Autodesk Fusion 360 part; units mm, degrees
(part 2 of 2)
extrude "Extrude1'" add sketch "clean_plate_v4.1" along normal blind 3 separate body contours L0 L1 L2 L3 L4 L5 A0 L29 L30 L33 L34 L36 L39 L40 L42 L43 L44 L46 L50 L51 L52 L53 L54 A2 L281 A12 L282 L283 L367 L368 L369 L370 A16 L371 L373 L374 L375 L377 L378 L379 L380 L381 L382 L383 L384 L386 L387 L390 L391 L392 L393 L395 L396 A17 L398 L399 L400 L403 L404 | L6 L7 L28 L31 L32 L41 A1 L64 L72 A4 L124 L126 L131 L133 L135 L136 L141 L142 L143 L144 L151 L154 L155 L157 L159 L160 L161 L166 L167 L169 L170 L171 L173 L174 L179 L181 L184 L185 L187 L188 L190 L192 L194 L195 L198 L200 L201 L204 L205 L208 L210 L215 L219 L225 L231 A13 A14 A15 | L8 L9 L15 L27 | L10 L12 L17 L21 | L11 L23 L24 L25 | L13 L14 L385 L397 | L16 L18 L19 L22 | L20 L127 L148 L156 | L26 L97 L115 L120 | L35 L376 L401 L402 | L37 L45 L49 L394 | L38 L55 L372 L389 | L47 L48 L56 L388 | L57 L74 L77 L363 | L58 L81 L355 L364 | L59 L253 L254 L257 | L60 L68 L91 L366 | L61 L65 L308 L310 | L62 L69 L80 L365 | L63 L246 L252 L256 | L66 L73 L82 L306 | L67 L70 L79 L85 | A3 | A9 | A7 | A5 | L260 L261 L262 L263 L264 L265 L267 L270 L274 L275 L276 L277 L278 L279 L280 L284 L285 L286 L287 L288 L289 L290 L291 L292 L293 L294 L295 L297 L298 L300 L301 L303 L304 L309 L311 L312 L314 L316 L318 L319 L321 L322 L323 L324 L325 L327 L329 L330 L331 L332 L335 L337 L338 L339 L342 L343 L345 L347 | L71 L75 L88 L353 | L76 L78 L83 L350 | L84 L86 L87 L90 | L89 L92 L357 L358 | L93 L94 L103 L104 | L95 L129 L130 L139 | L96 L106 L113 L116 | L98 L99 L102 L117 | L100 L108 L111 L118 | L101 L112 L121 L122 | L105 L107 L110 L114 | L109 L128 L137 L153 | L119 L123 L132 L140 | L125 L134 L180 L189 | L138 L147 L150 L152 | L145 L146 L149 L269 | L158 L175 L202 L207 | L162 L224 L227 L232 | L163 L177 L199 L221 | L164 L165 L172 L182 | L168 L209 L212 L214 | L176 L196 L213 L217 | L178 L211 L216 L230 | L183 L186 L191 L203 | L193 L206 L218 L226 | L197 L220 L222 L223 | L228 L229 L233 L237 | L234 L247 L248 L249 | L235 L236 L238 L250 | L239 L240 L241 L242 | L243 L244 L245 L251 | L255 L258 L259 L305 | L266 L326 L334 L346 | L268 L271 L272 L273 | L296 L317 L320 L340 | L299 L315 L336 L341 | L302 L328 L333 L344 | L307 L313 L356 L362 | L348 L351 L359 L361 | L349 L352 L354 L360 makes body 2 in component "bottom_right"
extrude "Extrude2'" cut sketch "clean_plate_v4.1" along normal blind 10 contours L0 L1 L2 L3 L4 L5 A0 L29 L30 L33 L34 L36 L39 L40 L42 L43 L44 L46 L50 L51 L52 L53 L54 A2 L281 A12 L282 L283 L367 L368 L369 L370 A16 L371 L373 L374 L375 L377 L378 L379 L380 L381 L382 L383 L384 L386 L387 L390 L391 L392 L393 L395 L396 A17 L398 L399 L400 L403 L404 | L6 L7 L28 L31 L32 L41 A1 L64 L72 A4 L124 L126 L131 L133 L135 L136 L141 L142 L143 L144 L151 L154 L155 L157 L159 L160 L161 L166 L167 L169 L170 L171 L173 L174 L179 L181 L184 L185 L187 L188 L190 L192 L194 L195 L198 L200 L201 L204 L205 L208 L210 L215 L219 L225 L231 A13 A14 A15 | A3 | A9 | A7 | A5 bodies 2 in component "bottom_right"
extrude "Extrude3'" add sketch "clean_plate_v4.1" along normal blind 10 contours L0 L1 L2 L3 L4 L5 A0 L29 L30 L33 L34 L36 L39 L40 L42 L43 L44 L46 L50 L51 L52 L53 L54 A2 L281 A12 L282 L283 L367 L368 L369 L370 A16 L371 L373 L374 L375 L377 L378 L379 L380 L381 L382 L383 L384 L386 L387 L390 L391 L392 L393 L395 L396 A17 L398 L399 L400 L403 L404 | L6 L7 L28 L31 L32 L41 A1 L64 L72 A4 L124 L126 L131 L133 L135 L136 L141 L142 L143 L144 L151 L154 L155 L157 L159 L160 L161 L166 L167 L169 L170 L171 L173 L174 L179 L181 L184 L185 L187 L188 L190 L192 L194 L195 L198 L200 L201 L204 L205 L208 L210 L215 L219 L225 L231 A13 A14 A15 | A3 | A9 | A7 | A5 bodies 2 in component "bottom_right"
extrude "Extrude4" cut sketch "clean_plate_v4.1" along normal blind 10 contours L0 L1 L2 L3 L4 L5 A0 L29 L30 L33 L34 L36 L39 L40 L42 L43 L44 L46 L50 L51 L52 L53 L54 A2 L281 A12 L282 L283 L367 L368 L369 L370 A16 L371 L373 L374 L375 L377 L378 L379 L380 L381 L382 L383 L384 L386 L387 L390 L391 L392 L393 L395 L396 A17 L398 L399 L400 L403 L404 | A3 | A9 | A7 | A5 bodies 2 makes body 3 at (77.3381, -75.3022, 10) in component "bottom_right"
extrude "Extrude5" add sketch "clean_plate_v4.1" along normal blind 7 contours L0 L1 L2 L3 L4 L5 A0 L29 L30 L33 L34 L36 L39 L40 L42 L43 L44 L46 L50 L51 L52 L53 L54 A2 L281 A12 L282 L283 L367 L368 L369 L370 A16 L371 L373 L374 L375 L377 L378 L379 L380 L381 L382 L383 L384 L386 L387 L390 L391 L392 L393 L395 L396 A17 L398 L399 L400 L403 L404 | A3 | A9 | A7 | A5 bodies 2 3 in component "bottom_right"
sketch "clean_plate_v4.1 (2)" plane through (0, 0, 0) normal (0, 0, 1) x (1, 0, 0) in component "top_left"
  line L0 (78.2004, -36.6162) -> (78.2605, -36.027)
  line L1 (224.705, -44.1568) -> (224.705, -44.9557)
  line L2 (78.2605, -36.027) -> (78.4684, -35.3561)
  line L3 (79.2324, -34.2221) -> (79.7595, -33.7872)
  arc A0 (179.1936, -126.194) -> (177.1936, -128.1938) centre (179.1936, -128.194) ccw
  line L4 (78.4684, -35.3561) -> (78.798, -34.7487)
  line L5 (78.798, -34.7487) -> (79.2324, -34.2221)
  line L6 (79.7595, -33.7872) -> (80.3665, -33.4582)
  line L7 (80.3665, -33.4582) -> (81.0392, -33.2493)
  line L8 (174.6938, -126.6937) -> (174.693, -134.5617)
  line L9 (98.7866, -145.4708) -> (98.354, -145.6898)
  line L10 (81.6298, -33.1903) -> (171.891, -33.187)
  line L11 (96.953, -145.9308) -> (96.1686, -145.7726)
  line L12 (80.8467, -125.7147) -> (77.5111, -119.9268)
  line L13 (75.6971, -41.0327) -> (75.7005, -36.4881)
  line L14 (224.705, -62.8443) -> (224.705, -102.1057)
  line L15 (171.891, -33.187) -> (218.5412, -40.2054)
  line L16 (78.1951, -43.6543) -> (78.2004, -36.6162)
  line L17 (81.0392, -33.2493) -> (81.6298, -33.1903)
  line L18 (92.4734, -145.8895) -> (89.7788, -141.2137)
  line L19 (75.6449, -110.7467) -> (75.6837, -58.9213)
  arc A1 (222.205, -104.7254) -> (222.205, -117.3746) centre (223.705, -111.05) cw
  line L20 (101.0994, -115.1193) -> (87.243, -123.1193)
  line L21 (98.354, -145.6898) -> (97.7123, -145.8798)
  line L22 (222.205, -44.5066) -> (222.205, -47.5754)
  line L23 (171.498, -138.3375) -> (170.8165, -138.405)
  arc A2 (177.6938, -123.694) -> (174.6938, -126.6937) centre (177.6938, -126.694) ccw
  line L24 (221.5253, -121.9381) -> (221.0349, -122.5329)
  line L25 (221.0885, -41.8996) -> (221.8203, -43.1589)
  line L26 (170.8165, -138.405) -> (110.9915, -138.405)
  line L27 (169.95, -115.8) -> (153.95, -115.8)
  line L28 (172.2545, -138.1006) -> (171.498, -138.3375)
  line L29 (174.6225, -135.2197) -> (174.3886, -135.9665)
  line L30 (96.1686, -145.7726) -> (95.4672, -145.4279)
  line L31 (174.0203, -136.6471) -> (173.5299, -137.2419)
  line L32 (221.8955, -121.2539) -> (221.5253, -121.9381)
  line L33 (174.693, -134.5617) -> (174.6225, -135.2197)
  line L34 (221.8203, -43.1589) -> (222.205, -44.5066)
  line L35 (94.9201, -144.9603) -> (94.5516, -144.4887)
  line L36 (218.5412, -40.2054) -> (219.9033, -40.8617)
  line L37 (219.7584, -123.3922) -> (218.9873, -123.6328)
  line L38 (94.5516, -144.4887) -> (90.6367, -137.6956)
  arc A3 (222.205, -47.5754) -> (222.205, -60.2246) centre (223.705, -53.9) cw
  arc A4 (90.6367, -137.6956) -> (84.3208, -126.7362) centre (86.1791, -132.9649) cw
  line L39 (78.7161, -115.942) -> (78.4204, -114.4636)
  line L40 (222.205, -117.3746) -> (222.205, -119.8357)
  line L41 (134.898, -116.828) -> (134.898, -132.828)
  line L42 (131.85, -134.2) -> (131.85, -118.2)
  line L43 (109.0994, -128.9757) -> (101.0994, -115.1193)
  line L44 (173.5299, -137.2419) -> (172.9351, -137.7323)
  line L45 (150.898, -132.828) -> (150.898, -116.828)
  line L46 (84.3208, -126.7362) -> (79.7448, -118.7959)
  line L47 (115.85, -118.2) -> (115.85, -134.2)
  line L48 (153.95, -131.8) -> (169.95, -131.8)
  line L49 (79.7448, -118.7959) -> (79.0518, -117.2209)
  line L50 (219.9033, -40.8617) -> (221.0885, -41.8996)
  line L51 (110.9915, -138.405) -> (98.7866, -145.4708)
  line L52 (172.9351, -137.7323) -> (172.2545, -138.1006)
  line L53 (95.243, -136.9757) -> (109.0994, -128.9757)
  line L54 (222.1218, -120.5231) -> (221.8955, -121.2539)
  line L55 (220.4401, -123.0233) -> (219.7584, -123.3922)
  line L56 (169.95, -131.8) -> (169.95, -115.8)
  line L57 (87.243, -123.1193) -> (95.243, -136.9757)
  line L58 (218.2905, -123.694) -> (177.6938, -123.694)
  line L59 (78.2135, -111.9846) -> (78.145, -110.6818)
  line L60 (78.145, -110.6818) -> (78.1857, -56.3034)
  line L61 (222.205, -119.8357) -> (222.1218, -120.5231)
  line L62 (222.205, -60.2246) -> (222.205, -104.7254)
  line L63 (79.0518, -117.2209) -> (78.7161, -115.942)
  line L64 (221.0349, -122.5329) -> (220.4401, -123.0233)
  line L65 (78.4204, -114.4636) -> (78.2803, -112.8531)
  arc A5 (78.1857, -56.3034) -> (78.1951, -43.6543) centre (76.6904, -49.9778) cw
  line L66 (218.9873, -123.6328) -> (218.2905, -123.694)
  line L67 (134.898, -132.828) -> (150.898, -132.828)
  line L68 (78.2803, -112.8531) -> (78.2135, -111.9846)
  line L69 (115.85, -134.2) -> (131.85, -134.2)
  line L70 (97.7123, -145.8798) -> (96.953, -145.9308)
  line L71 (174.3886, -135.9665) -> (174.0203, -136.6471)
  line L72 (131.85, -118.2) -> (115.85, -118.2)
  line L73 (95.4672, -145.4279) -> (94.9201, -144.9603)
  line L74 (150.898, -116.828) -> (134.898, -116.828)
  line L75 (153.95, -115.8) -> (153.95, -131.8)
  circle A6 centre (86.1791, -132.9649) radius 2
  line L76 (93.1049, -146.6975) -> (92.4734, -145.8895)
  line L77 (85.03, -71.09) -> (98.23, -71.09)
  line L78 (224.705, -119.9864) -> (224.5766, -121.0472)
  circle A7 centre (223.705, -111.05) radius 2
  line L79 (107.4, -62.05) -> (107.4, -76.05)
  line L80 (159.5, -91.31) -> (159.5, -77.31)
  line L81 (107.4, -57) -> (121.4, -57)
  line L82 (130.85, -133.2) -> (130.85, -119.2)
  line L83 (98.23, -71.09) -> (98.23, -40.39)
  line L84 (176.1036, -138.0502) -> (175.3059, -139.0179)
  line L85 (178.55, -111.75) -> (178.55, -97.75)
  circle A8 centre (76.6904, -49.9778) radius 2
  line L86 (224.5766, -121.0472) -> (224.2111, -122.2279)
  line L87 (121.4, -76.05) -> (121.4, -62.05)
  circle A9 centre (223.705, -53.9) radius 2
  line L88 (218.4, -126.194) -> (179.1936, -126.194)
  line L89 (76.6839, -118.0469) -> (76.2792, -116.505)
  line L90 (107.4, -76.05) -> (121.4, -76.05)
  line L91 (121.4, -62.05) -> (107.4, -62.05)
  line L92 (99.2811, -148.0225) -> (98.1564, -148.3556)
  circle A10 centre (223.705, -111.05) radius 4
  line L93 (80.5392, -30.7868) -> (81.5052, -30.6903)
  line L94 (75.7987, -35.5252) -> (76.1534, -34.3806)
  line L95 (172.0779, -30.687) -> (219.2863, -37.7893)
  line L96 (116.85, -119.2) -> (116.85, -133.2)
  line L97 (94.0822, -147.5328) -> (93.1049, -146.6975)
  line L98 (75.9418, -114.8181) -> (75.7886, -113.0573)
  line L99 (221.2947, -38.757) -> (223.044, -40.2889)
  line L100 (145.5, -77.31) -> (145.5, -91.31)
  line L101 (145.5, -91.31) -> (159.5, -91.31)
  line L102 (76.7158, -33.3442) -> (77.4564, -32.4462)
  line L103 (75.7005, -36.4881) -> (75.7987, -35.5252)
  line L104 (219.2863, -37.7893) -> (221.2947, -38.757)
  line L105 (81.5052, -30.6903) -> (172.0779, -30.687)
  line L106 (173.2321, -140.4142) -> (171.9999, -140.8)
  line L107 (99.9784, -147.6695) -> (99.2811, -148.0225)
  line L108 (77.4564, -32.4462) -> (78.3553, -31.7047)
  line L109 (224.2111, -122.2279) -> (223.6086, -123.3412)
  line L110 (178.55, -97.75) -> (164.55, -97.75)
  line L111 (171.9999, -140.8) -> (170.9399, -140.905)
  line L112 (177.1936, -128.1938) -> (177.193, -134.6953)
  line L113 (223.6086, -123.3412) -> (222.8109, -124.3089)
  line L114 (111.6629, -140.905) -> (99.9784, -147.6695)
  line L115 (159.5, -77.31) -> (145.5, -77.31)
  line L116 (174.3382, -139.8156) -> (173.2321, -140.4142)
  line L117 (107.4, -43) -> (107.4, -57)
  line L118 (121.4, -57) -> (121.4, -43)
  line L119 (85.03, -40.39) -> (85.03, -71.09)
  circle A11 centre (76.6904, -49.9778) radius 4
  line L120 (170.9399, -140.905) -> (111.6629, -140.905)
  line L121 (98.1564, -148.3556) -> (96.7866, -148.4476)
  circle A12 centre (223.705, -53.9) radius 4
  line L122 (176.7022, -136.9441) -> (176.1036, -138.0502)
  line L123 (130.85, -119.2) -> (116.85, -119.2)
  line L124 (75.7886, -113.0573) -> (75.7186, -112.1461)
  line L125 (76.2792, -116.505) -> (75.9418, -114.8181)
  line L126 (75.7186, -112.1461) -> (75.6449, -110.7467)
  line L127 (96.7866, -148.4476) -> (95.3567, -148.1592)
  line L128 (149.898, -131.828) -> (149.898, -117.828)
  line L129 (140.45, -54.6) -> (140.45, -40.6)
  line L130 (140.45, -59.65) -> (126.45, -59.65)
  line L131 (145.5, -72.26) -> (159.5, -72.26)
  line L132 (216.65, -85) -> (202.65, -85)
  line L133 (216.65, -46.9) -> (202.65, -46.9)
  line L134 (126.45, -59.65) -> (126.45, -73.65)
  line L135 (159.5, -58.26) -> (145.5, -58.26)
  line L136 (140.45, -92.7) -> (140.45, -78.7)
  line L137 (178.55, -73.65) -> (178.55, -59.65)
  line L138 (178.55, -59.65) -> (164.55, -59.65)
  line L139 (197.6, -78.45) -> (197.6, -64.45)
  line L140 (177.082, -135.7313) -> (176.7022, -136.9441)
  line L141 (164.55, -73.65) -> (178.55, -73.65)
  line L142 (197.6, -64.45) -> (183.6, -64.45)
  line L143 (79.3908, -31.1434) -> (80.5392, -30.7868)
  line L144 (135.898, -117.828) -> (135.898, -131.828)
  line L145 (126.45, -54.6) -> (140.45, -54.6)
  line L146 (126.45, -78.7) -> (126.45, -92.7)
  line L147 (83.4748, -105.2852) -> (97.4748, -105.2852)
  line L148 (160.5, -92.31) -> (160.5, -76.31)
  line L149 (121.4, -43) -> (107.4, -43)
  line L150 (178.55, -54.6) -> (178.55, -40.6)
  line L151 (178.55, -40.6) -> (164.55, -40.6)
  line L152 (159.5, -72.26) -> (159.5, -58.26)
  line L153 (202.65, -85) -> (202.65, -99)
  line L154 (222.8109, -124.3089) -> (221.8432, -125.1066)
  line L155 (224.1387, -42.1727) -> (224.705, -44.1568)
  line L156 (149.898, -117.828) -> (135.898, -117.828)
  line L157 (164.55, -40.6) -> (164.55, -54.6)
  line L158 (121.4, -100.15) -> (107.4, -100.15)
  line L159 (107.4, -114.15) -> (121.4, -114.15)
  line L160 (175.3059, -139.0179) -> (174.3382, -139.8156)
  line L161 (107.4, -100.15) -> (107.4, -114.15)
  line L162 (98.23, -40.39) -> (85.03, -40.39)
  line L163 (121.4, -114.15) -> (121.4, -100.15)
  line L164 (140.45, -40.6) -> (126.45, -40.6)
  line L165 (126.45, -92.7) -> (140.45, -92.7)
  line L166 (220.7348, -125.7064) -> (219.4745, -126.0997)
  line L167 (164.55, -111.75) -> (178.55, -111.75)
  line L168 (116.85, -133.2) -> (130.85, -133.2)
  line L169 (95.3567, -148.1592) -> (94.0822, -147.5328)
  line L170 (76.1534, -34.3806) -> (76.7158, -33.3442)
  line L171 (164.55, -54.6) -> (178.55, -54.6)
  line L172 (219.4745, -126.0997) -> (218.4, -126.194)
  line L173 (202.65, -46.9) -> (202.65, -60.9)
  line L174 (126.45, -73.65) -> (140.45, -73.65)
  line L175 (164.55, -97.75) -> (164.55, -111.75)
  line L176 (202.65, -60.9) -> (216.65, -60.9)
  line L177 (216.65, -99) -> (216.65, -85)
  line L178 (202.65, -99) -> (216.65, -99)
  line L179 (216.65, -60.9) -> (216.65, -46.9)
  line L180 (140.45, -78.7) -> (126.45, -78.7)
  line L181 (140.45, -73.65) -> (140.45, -59.65)
  line L182 (126.45, -40.6) -> (126.45, -54.6)
  line L183 (223.044, -40.2889) -> (224.1387, -42.1727)
  line L184 (145.5, -58.26) -> (145.5, -72.26)
  line L185 (77.5111, -119.9268) -> (76.6839, -118.0469)
  line L186 (164.55, -59.65) -> (164.55, -73.65)
  line L187 (221.8432, -125.1066) -> (220.7348, -125.7064)
  line L188 (135.898, -131.828) -> (149.898, -131.828)
  line L189 (177.193, -134.6953) -> (177.082, -135.7313)
  line L190 (198.6, -98.5) -> (198.6, -82.5)
  line L191 (183.6, -78.45) -> (197.6, -78.45)
  line L192 (141.45, -77.7) -> (125.45, -77.7)
  line L193 (163.55, -93.7) -> (179.55, -93.7)
  line L194 (144.5, -92.31) -> (160.5, -92.31)
  line L195 (183.6, -64.45) -> (183.6, -78.45)
  arc A13 (224.705, -62.8443) -> (224.705, -44.9557) centre (223.705, -53.9) ccw
  line L196 (197.6, -97.5) -> (197.6, -83.5)
  arc A14 (75.6971, -41.0327) -> (75.6837, -58.9213) centre (76.6904, -49.9778) ccw
  line L197 (179.55, -74.65) -> (179.55, -58.65)
  line L198 (201.65, -64.95) -> (201.65, -80.95)
  line L199 (197.6, -83.5) -> (183.6, -83.5)
  line L200 (183.6, -97.5) -> (197.6, -97.5)
  line L201 (183.6, -83.5) -> (183.6, -97.5)
  line L202 (163.55, -77.7) -> (163.55, -93.7)
  line L203 (179.55, -77.7) -> (163.55, -77.7)
  line L204 (159.5, -96.36) -> (145.5, -96.36)
  line L205 (141.45, -93.7) -> (141.45, -77.7)
  line L206 (144.5, -95.36) -> (144.5, -111.36)
  line L207 (160.5, -95.36) -> (144.5, -95.36)
  line L208 (201.65, -103.05) -> (201.65, -119.05)
  line L209 (97.4748, -91.2851) -> (83.4748, -91.2851)
  line L210 (159.5, -110.36) -> (159.5, -96.36)
  line L211 (182.6, -101.55) -> (182.6, -117.55)
  line L212 (201.65, -119.05) -> (217.65, -119.05)
  line L213 (198.6, -82.5) -> (182.6, -82.5)
  line L214 (217.65, -100) -> (217.65, -84)
  line L215 (97.4748, -105.2852) -> (97.4748, -91.2851)
  line L216 (122.4, -80.1) -> (106.4, -80.1)
  line L217 (182.6, -82.5) -> (182.6, -98.5)
  line L218 (145.5, -96.36) -> (145.5, -110.36)
  line L219 (197.6, -102.55) -> (183.6, -102.55)
  arc A15 (224.704, -119.9944) -> (224.705, -102.1057) centre (223.705, -111.05) ccw
  circle A16 centre (86.1791, -132.9649) radius 4
  line L220 (163.55, -58.65) -> (163.55, -74.65)
  line L221 (125.45, -93.7) -> (141.45, -93.7)
  line L222 (179.55, -58.65) -> (163.55, -58.65)
  arc A17 (80.8467, -125.7147) -> (89.7788, -141.2137) centre (86.1791, -132.9649) ccw
  line L223 (163.55, -74.65) -> (179.55, -74.65)
  line L224 (197.6, -116.55) -> (197.6, -102.55)
  line L225 (183.6, -116.55) -> (197.6, -116.55)
  line L226 (78.3553, -31.7047) -> (79.3908, -31.1434)
  line L227 (83.4748, -91.2851) -> (83.4748, -105.2852)
  line L228 (145.5, -110.36) -> (159.5, -110.36)
  line L229 (179.55, -93.7) -> (179.55, -77.7)
  line L230 (125.45, -77.7) -> (125.45, -93.7)
  line L231 (183.6, -102.55) -> (183.6, -116.55)
  line L232 (144.5, -76.31) -> (144.5, -92.31)
  line L233 (182.6, -98.5) -> (198.6, -98.5)
  line L234 (160.5, -76.31) -> (144.5, -76.31)
  line L235 (81.0083, -35.9979) -> (81.1637, -35.8697)
  line L236 (171.704, -35.687) -> (217.796, -42.6214)
  line L237 (218.512, -42.9664) -> (219.133, -43.5102)
  line L238 (219.133, -43.5102) -> (219.502, -44.1452)
  line L239 (163.55, -112.75) -> (179.55, -112.75)
  line L240 (80.7223, -36.5288) -> (80.7834, -36.3316)
  line L241 (81.5392, -35.7118) -> (81.7544, -35.6903)
  line L242 (217.796, -42.6214) -> (218.512, -42.9664)
  line L243 (182.6, -117.55) -> (198.6, -117.55)
  line L244 (160.5, -73.26) -> (160.5, -57.26)
  line L245 (125.45, -112.75) -> (141.45, -112.75)
  line L246 (141.45, -112.75) -> (141.45, -96.75)
  line L247 (198.6, -117.55) -> (198.6, -101.55)
  line L248 (144.5, -73.26) -> (160.5, -73.26)
  line L249 (160.5, -57.26) -> (144.5, -57.26)
  line L250 (106.4, -115.15) -> (122.4, -115.15)
  line L251 (217.65, -119.05) -> (217.65, -103.05)
  line L252 (182.6, -79.45) -> (198.6, -79.45)
  line L253 (80.8802, -36.1532) -> (81.0083, -35.9979)
  line L254 (144.5, -57.26) -> (144.5, -73.26)
  line L255 (217.65, -64.95) -> (201.65, -64.95)
  line L256 (160.5, -111.36) -> (160.5, -95.36)
  line L257 (219.705, -119.685) -> (219.667, -119.999)
  line L258 (81.3421, -35.773) -> (81.5392, -35.7118)
  line L259 (80.7834, -36.3316) -> (80.8802, -36.1532)
  line L260 (219.667, -119.999) -> (219.58, -120.28)
  line L261 (219.502, -44.1452) -> (219.705, -44.8564)
  line L262 (80.7003, -36.7444) -> (80.7223, -36.5288)
  line L263 (219.705, -44.8564) -> (219.705, -119.685)
  line L264 (219.58, -120.28) -> (219.442, -120.535)
  line L265 (219.442, -120.535) -> (219.259, -120.757)
  line L266 (201.65, -80.95) -> (217.65, -80.95)
  line L267 (198.6, -101.55) -> (182.6, -101.55)
  line L268 (179.55, -96.75) -> (163.55, -96.75)
  line L269 (198.6, -79.45) -> (198.6, -63.45)
  line L270 (122.4, -96.1) -> (122.4, -80.1)
  line L271 (217.65, -80.95) -> (217.65, -64.95)
  line L272 (201.65, -100) -> (217.65, -100)
  line L273 (106.4, -96.1) -> (122.4, -96.1)
  line L274 (144.5, -111.36) -> (160.5, -111.36)
  line L275 (122.4, -99.15) -> (106.4, -99.15)
  line L276 (141.45, -96.75) -> (125.45, -96.75)
  line L277 (179.55, -112.75) -> (179.55, -96.75)
  line L278 (217.65, -84) -> (201.65, -84)
  line L279 (171.754, -135.466) -> (171.532, -135.649)
  line L280 (106.4, -99.15) -> (106.4, -115.15)
  line L281 (125.45, -96.75) -> (125.45, -112.75)
  line L282 (219.037, -120.94) -> (218.782, -121.078)
  line L283 (163.55, -96.75) -> (163.55, -112.75)
  line L284 (122.4, -115.15) -> (122.4, -99.15)
  line L285 (106.4, -80.1) -> (106.4, -96.1)
  line L286 (164.55, -78.7) -> (164.55, -92.7)
  line L287 (216.65, -79.95) -> (216.65, -65.95)
  line L288 (163.55, -39.6) -> (163.55, -55.6)
  line L289 (96.6298, -143.088) -> (81.9785, -117.665)
  line L290 (182.6, -63.45) -> (182.6, -79.45)
  line L291 (217.65, -103.05) -> (201.65, -103.05)
  line L292 (140.45, -111.75) -> (140.45, -97.75)
  line L293 (219.259, -120.757) -> (219.037, -120.94)
  line L294 (179.55, -55.6) -> (179.55, -39.6)
  line L295 (198.6, -63.45) -> (182.6, -63.45)
  line L296 (81.1637, -35.8697) -> (81.3421, -35.773)
  line L297 (179.55, -39.6) -> (163.55, -39.6)
  line L298 (218.5, -121.166) -> (218.181, -121.194)
  line L299 (170.693, -135.905) -> (110.32, -135.905)
  line L300 (201.65, -84) -> (201.65, -100)
  line L301 (81.7544, -35.6903) -> (171.704, -35.687)
  line L302 (81.153, -115.379) -> (80.899, -114.109)
  line L303 (172.817, -122.736) -> (172.494, -123.331)
  line L304 (202.65, -79.95) -> (216.65, -79.95)
  line L305 (216.65, -65.95) -> (202.65, -65.95)
  line L306 (122.4, -42) -> (106.4, -42)
  line L307 (96.7353, -143.223) -> (96.6298, -143.088)
  line L308 (171.937, -135.244) -> (171.754, -135.466)
  line L309 (140.45, -97.75) -> (126.45, -97.75)
  line L310 (173.762, -121.791) -> (173.244, -122.218)
  line L311 (163.55, -55.6) -> (179.55, -55.6)
  line L312 (172.194, -124.696) -> (172.193, -134.428)
  line L313 (106.4, -42) -> (106.4, -58)
  line L314 (172.193, -134.428) -> (172.163, -134.708)
  line L315 (172.29, -123.988) -> (172.194, -124.696)
  line L316 (173.244, -122.218) -> (172.817, -122.736)
  line L317 (107.4, -95.1) -> (121.4, -95.1)
  line L318 (175.014, -121.265) -> (174.356, -121.468)
  line L319 (122.4, -58) -> (122.4, -42)
  line L320 (106.4, -58) -> (122.4, -58)
  line L321 (145.5, -39.21) -> (145.5, -53.21)
  line L322 (145.5, -53.21) -> (159.5, -53.21)
  line L323 (81.9785, -117.665) -> (81.4197, -116.395)
  line L324 (126.45, -111.75) -> (140.45, -111.75)
  line L325 (171.277, -135.787) -> (170.996, -135.875)
  line L326 (121.4, -95.1) -> (121.4, -81.1)
  line L327 (164.55, -92.7) -> (178.55, -92.7)
  line L328 (107.4, -81.1) -> (107.4, -95.1)
  line L329 (172.075, -134.989) -> (171.937, -135.244)
  line L330 (80.899, -114.109) -> (80.772, -112.649)
  line L331 (218.782, -121.078) -> (218.5, -121.166)
  line L332 (126.45, -97.75) -> (126.45, -111.75)
  line L333 (97.1193, -143.414) -> (96.9805, -143.386)
  line L334 (202.65, -65.95) -> (202.65, -79.95)
  line L335 (80.7085, -111.823) -> (80.645, -110.617)
  line L336 (97.5948, -143.272) -> (97.4269, -143.357)
  line L337 (172.494, -123.331) -> (172.29, -123.988)
  line L338 (97.2682, -143.404) -> (97.1193, -143.414)
  line L339 (172.163, -134.708) -> (172.075, -134.989)
  line L340 (174.356, -121.468) -> (173.762, -121.791)
  line L341 (170.996, -135.875) -> (170.693, -135.905)
  line L342 (97.4269, -143.357) -> (97.2682, -143.404)
  line L343 (175.719, -121.194) -> (175.014, -121.265)
  line L344 (141.45, -74.65) -> (141.45, -58.65)
  line L345 (197.6, -45.4) -> (183.6, -45.4)
  line L346 (80.645, -110.617) -> (80.7003, -36.7444)
  line L347 (122.4, -77.05) -> (122.4, -61.05)
  line L348 (202.65, -104.05) -> (202.65, -118.05)
  line L349 (125.45, -55.6) -> (141.45, -55.6)
  line L350 (171.532, -135.649) -> (171.277, -135.787)
  line L351 (218.181, -121.194) -> (175.719, -121.194)
  line L352 (121.4, -81.1) -> (107.4, -81.1)
  line L353 (96.8523, -143.323) -> (96.7353, -143.223)
  line L354 (144.5, -54.21) -> (160.5, -54.21)
  line L355 (182.6, -60.4) -> (198.6, -60.4)
  line L356 (178.55, -92.7) -> (178.55, -78.7)
  line L357 (81.4197, -116.395) -> (81.153, -115.379)
  line L358 (96.9805, -143.386) -> (96.8523, -143.323)
  line L359 (80.772, -112.649) -> (80.7085, -111.823)
  line L360 (198.6, -44.4) -> (182.6, -44.4)
  line L361 (178.55, -78.7) -> (164.55, -78.7)
  line L362 (159.5, -53.21) -> (159.5, -39.21)
  line L363 (110.32, -135.905) -> (97.5948, -143.272)
  line L364 (160.5, -38.21) -> (144.5, -38.21)
  line L365 (183.6, -59.4) -> (197.6, -59.4)
  line L366 (141.45, -58.65) -> (125.45, -58.65)
  line L367 (141.45, -55.6) -> (141.45, -39.6)
  line L368 (95.23, -43.39) -> (88.03, -43.39)
  line L369 (88.03, -68.09) -> (95.23, -68.09)
  line L370 (141.45, -39.6) -> (125.45, -39.6)
  line L371 (168.95, -130.8) -> (168.95, -116.8)
  line L372 (95.23, -68.09) -> (95.23, -43.39)
  line L373 (201.65, -45.9) -> (201.65, -61.9)
  line L374 (88.03, -43.39) -> (88.03, -68.09)
  line L375 (217.65, -45.9) -> (201.65, -45.9)
  line L376 (198.6, -60.4) -> (198.6, -44.4)
  line L377 (122.4, -61.05) -> (106.4, -61.05)
  line L378 (160.5, -54.21) -> (160.5, -38.21)
  line L379 (159.5, -39.21) -> (145.5, -39.21)
  line L380 (107.7334, -128.6097) -> (100.7334, -116.4853)
  line L381 (98.4748, -90.2851) -> (82.4748, -90.2851)
  line L382 (100.7334, -116.4853) -> (88.609, -123.4853)
  line L383 (82.4748, -106.2852) -> (98.4748, -106.2852)
  line L384 (125.45, -39.6) -> (125.45, -55.6)
  line L385 (197.6, -59.4) -> (197.6, -45.4)
  line L386 (88.609, -123.4853) -> (95.609, -135.6097)
  line L387 (106.4, -77.05) -> (122.4, -77.05)
  line L388 (125.45, -74.65) -> (141.45, -74.65)
  line L389 (95.609, -135.6097) -> (107.7334, -128.6097)
  line L390 (216.65, -104.05) -> (202.65, -104.05)
  line L391 (183.6, -45.4) -> (183.6, -59.4)
  line L392 (168.95, -116.8) -> (154.95, -116.8)
  line L393 (82.4748, -90.2851) -> (82.4748, -106.2852)
  line L394 (216.65, -118.05) -> (216.65, -104.05)
  line L395 (154.95, -130.8) -> (168.95, -130.8)
  line L396 (98.4748, -106.2852) -> (98.4748, -90.2851)
  line L397 (106.4, -61.05) -> (106.4, -77.05)
  line L398 (144.5, -38.21) -> (144.5, -54.21)
  line L399 (154.95, -116.8) -> (154.95, -130.8)
  line L400 (201.65, -61.9) -> (217.65, -61.9)
  line L401 (125.45, -58.65) -> (125.45, -74.65)
  line L402 (217.65, -61.9) -> (217.65, -45.9)
  line L403 (202.65, -118.05) -> (216.65, -118.05)
  line L404 (182.6, -44.4) -> (182.6, -60.4)
extrude "Extrude1''" add sketch "clean_plate_v4.1 (2)" along normal blind 3 separate body contours L0 L2 L3 L4 L5 L6 L7 L8 L9 L10 L11 L15 L16 L17 A1 L21 L22 L23 A2 L24 L25 L26 L28 L29 L30 L31 L32 L33 L34 L35 L36 L37 L38 A3 A4 L39 L40 L44 L46 L49 L50 L51 L52 L54 L55 L58 L59 L60 L61 L62 L63 L64 L65 A5 L66 L68 L70 L71 L73 | L1 A0 L12 L13 L14 L18 L19 L76 L78 L84 L86 L88 L89 L92 L93 L94 L95 L97 L98 L99 L102 L103 L104 L105 L106 L107 L108 L109 L111 L112 L113 L114 L116 L120 L121 L122 L124 L125 L126 L127 L140 L143 L154 L155 L160 L166 L169 L170 L172 L183 L185 L187 L189 A13 A14 A15 A17 L226 | A10 | A16 | A11 | A12 makes body 4 in component "top_left"
extrude "Extrude2''" add sketch "clean_plate_v4.1 (2)" along normal blind 5 separate body contours L1 A0 L12 L13 L14 L18 L19 L76 L78 L84 L86 L88 L89 L92 L93 L94 L95 L97 L98 L99 L102 L103 L104 L105 L106 L107 L108 L109 L111 L112 L113 L114 L116 L120 L121 L122 L124 L125 L126 L127 L140 L143 L154 L155 L160 L166 L169 L170 L172 L183 L185 L187 L189 A13 A14 A15 A17 L226 makes body 5 in component "top_left"
extrude "Extrude3''" add 1 faces at (77.3381, -75.3022, 5) along direction (0, 0, 1) blind 2 on bodies 5 bodies 5 in component "top_left"
extrude "Extrude4'" add 1 faces at (79.0064, -73.172, 3) along direction (0, 0, 1) blind 2 on bodies 4 bodies 4 5 in component "top_left"
extrude "Extrude5'" cut 1 faces at (77.3381, -75.3022, 7) along direction (0, 0, -1) blind 0.5 on bodies 4 bodies 4 in component "top_left"
extrude "Extrude6" cut 1 faces at (77.3381, -75.3022, 10) along direction (0, 0, -1) blind 1.5 on bodies 2 bodies 2 in component "bottom_right"
component "plate_left" placed x (1, 0, 0) y (0, 1, 0) z (0, 0, 1) at (0, 0, 0)
component "bottom_right" placed x (1, 0, 0) y (0, 1, 0) z (0, 0, 1) at (0, 0, 0)
component "top_left" placed x (1, 0, 0) y (0, 1, 0) z (0, 0, 1) at (0, 0, 0)
